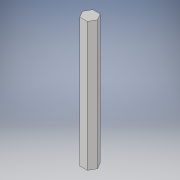
# Autodesk Inventor part: hex shaft for wheels
Saved by Autodesk Inventor 2019 (Build 230136000, 136)
## iProperties
Created: 2019-01-19
Part Number: hex shaft for wheels
Material: Generic
Document SubType Name: Modeling
Designer: Tiberus
Density: 1 g/cm^3
Appearance: Default
Author: Tiberus
Autodesk Inventor part; units mm, degrees
ref_plane "YZ Plane" through (0, 0, 0) normal (1, 0, 0) x (0, 1, 0)
ref_plane "XZ Plane" through (0, 0, 0) normal (0, 1, 0) x (-1, 0, 0)
ref_plane "XY Plane" through (0, 0, 0) normal (0, 0, 1) x (1, 0, 0)
sketch "Sketch1" plane through (0, 0, 0) normal (0, 1, 0) x (-1, 0, 0)
  line L0 (0, 0) -> (7.366, 0) construction
  line L1 (7.366, 0) -> (3.683, -6.3791)
  line L2 (3.683, -6.3791) -> (-3.683, -6.3791)
  line L3 (-3.683, -6.3791) -> (-7.366, 0)
  line L4 (-7.366, 0) -> (-3.683, 6.3791)
  line L5 (-3.683, 6.3791) -> (3.683, 6.3791)
  line L6 (3.683, 6.3791) -> (7.366, 0)
  dimension "d3" = 7.366
  constraints: 14 end point, 2 coincident, 13 other
  measures "d3" distance of L1.end L2.end
extrude "Extrusion1" add sketch "Sketch1" along normal blind 127
body "Solid1"
